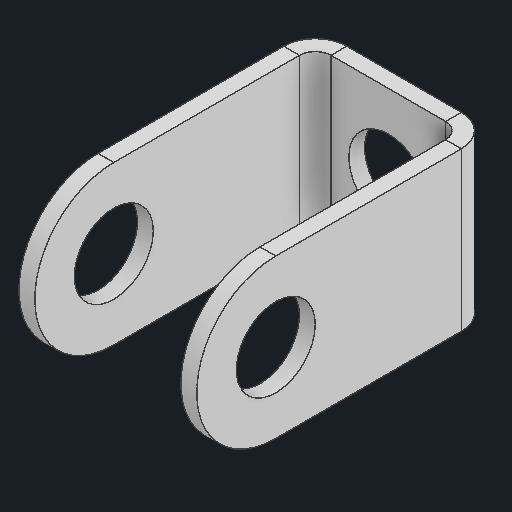
# Autodesk Inventor part: LA-T8-Bracket
Saved by Autodesk Inventor 2025.2 (Build 292293000, 293)
## iProperties
Created: 2025-08-15
Part Number: LA-T8-Bracket
Material: Generic
Document SubType Name: Sheet Metal
Designer: valer
Density: 1 g/cm^3
Sheet Metal Rule: Default_mm
Appearance: Default
Author: valer
Autodesk Inventor part; units mm, degrees
ref_plane "YZ Plane" through (0, 0, 0) normal (1, 0, 0) x (0, 1, 0)
ref_plane "XZ Plane" through (0, 0, 0) normal (0, 1, 0) x (-1, 0, 0)
ref_plane "XY Plane" through (0, 0, 0) normal (0, 0, 1) x (1, 0, 0)
sketch "Sketch1" plane through (0, 0, 0) normal (0, 0, 1) x (1, 0, 0)
  circle A0 centre (0, 0) radius 2
  line L0 (-4.5, 4) -> (4.5, 4)
  line L1 (4.5, 4) -> (4.5, -4)
  line L2 (4.5, -4) -> (-4.5, -4)
  line L3 (-4.5, -4) -> (-4.5, 4)
  line L4 (-4.5, 4) -> (4.5, -4) construction
  dimension "d0" = 4
  dimension "d1" = 8
  dimension "d2" = 9
  measures "d0" diameter of A0
  measures "d1" distance of L0.end L1.end
  measures "d2" distance of L0.start L0.end
extrude "Plate1" add sketch "Sketch1" along normal blind 0.8
sketch "Sketch2" plane through (3.7, 4, 0) normal (1, 0, 0) x (0, 1, 0)
  line L0 (-8, 0) -> (0, 0)
  line L1 (0, 0) -> (0, 15)
  line L2 (0, 15) -> (-8, 15)
  line L3 (-8, 15) -> (-8, 0)
  constraints: 6 end point, 1 horizontal, 1 perpendicular, 1 vertical
edge flange "Flange1" height 15 angle 90 thickness 0.8 bend radius 0.8 thickness toward (1, 0, 0) relief tear relief width 0.8 relief depth 0.4 corner gap 0.8 corner form 0 edges at (4.5, 0, 0.8) (-4.5, 0, 0.8) wall of the first edge with corners at (3.7, -4, 0) (3.7, 4, 0) (3.7, 4, 15) (3.7, -4, 15)
bend "Bend1"
corner "Corner1"
sketch "Sketch3" plane through (-4.5, -4, 15) normal (-1, 0, 0) x (0, 0, 1)
  line L0 (-13.4, 8) -> (-13.4, 0) construction
  line L1 (0, 0) -> (-13.4, 0) projected
  line L2 (0, 8) -> (0, 0) projected
  line L3 (-13.4, 8) -> (0, 8) projected
  circle A0 centre (-4, 4) radius 4
  point P0 (-15, 4)
  point P1 (-4, 8)
  point P2 (0, 4)
  point P3 (-4, 0)
  constraints: 3 tangent, 1 centre point
extrude "Cut1" cut sketch "Sketch3" against normal through all contours L1 A0 L2 | A0 L3 L2
sketch "Sketch4" plane through (-4.5, -4, 1.6) normal (-1, 0, 0) x (0, 0, 1)
  arc A0 (9.4, 0) -> (9.4, 8) centre (9.4, 4) ccw projected
  circle A1 centre (9.4, 4) radius 2
  point P0 (-1.6, 4)
  dimension "d16" = 4
  constraints: 1 centre point, 1 coincident
  measures "d16" diameter of A1
extrude "Cut2" cut sketch "Sketch4" against normal through all
equation "\"d14\" = Thickness"
equation "\"d17\" = Thickness"
equation "\"d3\" = Thickness"
equation "\"d4\" = BendReliefWidth"
equation "\"d5\" = BendReliefDepth"
equation "\"d6\" = MinimumRemnant"
equation "\"d7\" = TransitionRadius"
equation "\"d10\" = BendRadius"
equation "\"d11\" = CornerReliefSize"
equation "\"d12\" = GapSize"
equation "\"d13\" = JacobiRadiusSize"
equation "\"BendRadius\" = Thickness"
equation "\"BendReliefWidth\" = Thickness"
equation "\"BendReliefDepth\" = 0.5 * Thickness"
equation "\"CornerReliefSize\" = 4 * Thickness"
equation "\"MinimumRemnant\" = 2 * Thickness"
equation "\"TransitionRadius\" = BendRadius"
equation "\"JacobiRadiusSize\" = BendRadius"
equation "\"GapSize\" = Thickness"
equation "\"Thickness\" = 0.8"
body "Solid1"
